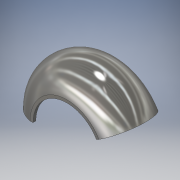
# Autodesk Inventor part: throwerRamp
Saved by Autodesk Inventor 2016 (Build 200138000, 138)
## iProperties
Created: 2015-11-01
Part Number: throwerRamp
Material: Generic
Document SubType Name: Modeling
Designer: rossmosier
Density: 1 g/cm^3
Appearance: Chrome - Polished Black
Author: rossmosier
Autodesk Inventor part; units mm, degrees
ref_plane "YZ Plane" through (0, 0, 0) normal (1, 0, 0) x (0, 1, 0)
ref_plane "XZ Plane" through (0, 0, 0) normal (0, 1, 0) x (-1, 0, 0)
ref_plane "XY Plane" through (0, 0, 0) normal (0, 0, 1) x (1, 0, 0)
sketch "Sketch2" plane through (0, 0, 0) normal (0, 1, 0) x (-1, 0, 0)
  line L0 (0, 0) -> (0, -107.95) construction
  line L1 (0, -53.975) -> (44.45, -53.975) construction
  arc A0 (0, -107.95) -> (0, 0) centre (-10.5455, -53.975) ccw
  arc A1 (0, -114.4073) -> (0, 6.4573) centre (-10.5455, -53.975) ccw
  line L2 (0, 0) -> (0, 6.4573)
  line L3 (0, -107.95) -> (0, -114.4073)
  line L4 (0, 6.4573) -> (-6.35, 6.4573)
  line L5 (-6.35, 6.4573) -> (-6.35, 0)
  line L6 (-6.35, 0) -> (0, 0)
  line L7 (0, 0) -> (0, 6.4573)
  line L8 (0, -107.95) -> (-6.35, -107.95)
  line L9 (-6.35, -107.95) -> (-6.35, -114.4073)
  line L10 (-6.35, -114.4073) -> (0, -114.4073)
  line L11 (0, -114.4073) -> (0, -107.95)
  line L12 (44.45, -53.975) -> (-82.55, -53.975) construction
  line L13 (-82.5742, -64.2808) -> (-82.5742, -44.6455) construction
  dimension "d5" = 107.95
  dimension "d6" = 44.45
  dimension "d7" = 6.35
  dimension "d8" = 6.35
  dimension "d9" = 127
  constraints: 28 end point, 5 point on circle, 4 horizontal, 4 parallel, 3 vertical, 2 centre point, 2 perpendicular, 2 point on line, 1 coincident, 1 midpoint
  measures "d5" distance of L0.start L0.end
  measures "d6" distance of L1.start L1.end
  measures "d7" radial gap between concentric circles of A0 A1
  measures "d8" distance of L6.end L5.end
  measures "d9" distance of L1.end L12.end
revolve "Revolution2" add sketch "Sketch2" angle 150 about axis through (82.5742, 0, -64.2808) along (0, 0, -1)
body "Solid3"
